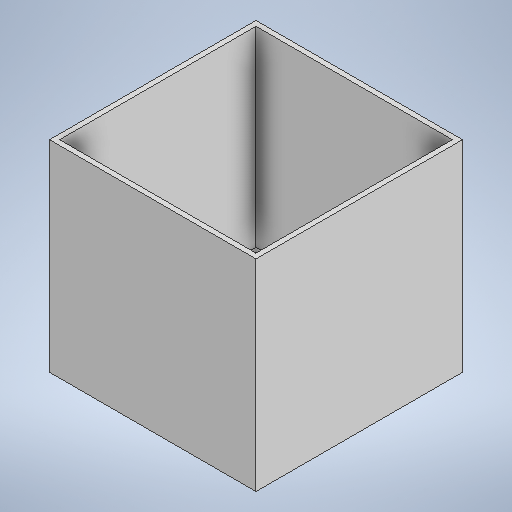
# Autodesk Inventor part: vaso
Saved by Autodesk Inventor 2025.1 (Build 291241000, 241)
## iProperties
Created: 2024-11-12
Part Number: vaso
Material: Genérico
Document SubType Name: Modeling
Designer: pedro
Density: 1 g/cm^3
Appearance: Padrão
Author: pedro
Autodesk Inventor part; units mm, degrees
ref_plane "YZ Plane" through (0, 0, 0) normal (1, 0, 0) x (0, 1, 0)
ref_plane "XZ Plane" through (0, 0, 0) normal (0, 1, 0) x (-1, 0, 0)
ref_plane "XY Plane" through (0, 0, 0) normal (0, 0, 1) x (1, 0, 0)
sketch "Esboço1" plane through (0, 0, 0) normal (0, 1, 0) x (-1, 0, 0)
  line L0 (102.5, 102.5) -> (-102.5, 102.5)
  line L1 (-102.5, 102.5) -> (-102.5, -102.5)
  line L2 (-102.5, -102.5) -> (102.5, -102.5)
  line L3 (102.5, -102.5) -> (102.5, 102.5)
  point P0 (0, 0)
  dimension "d0" = 205
  dimension "d1" = 205
  dimension "d2" = 102.5
  dimension "d3" = 102.5
  constraints: 8 end point, 2 parallel, 1 horizontal, 1 perpendicular
  measures "d0" distance of L2.end L1.end
  measures "d1" distance of L1.end L0.end
  measures "d2" distance from line of point (0, 0) L0
  measures "d3" distance from line of L3 point (0, 0)
extrude "Extrusão1" add sketch "Esboço1" along normal blind 200
sketch "Esboço2" plane through (0, 200, 0) normal (0, 1, 0) x (1, 0, 0)
  line L0 (-97.5, 97.5) -> (-97.5, -97.5)
  line L1 (-97.5, -97.5) -> (97.5, -97.5)
  line L2 (-97.5, 97.5) -> (97.5, 97.5)
  line L3 (97.5, 97.5) -> (97.5, -97.5)
  line L4 (-102.5, 102.5) -> (-102.5, -102.5) projected
  line L5 (102.5, 102.5) -> (-102.5, 102.5) projected
  line L6 (-102.5, -102.5) -> (102.5, -102.5) projected
  line L7 (102.5, -102.5) -> (102.5, 102.5) projected
  point P0 (0, 0)
  dimension "d6" = 5
  dimension "d7" = 5
  dimension "d8" = 5
  dimension "d9" = 5
  constraints: 8 end point, 2 perpendicular, 1 horizontal, 1 vertical
  measures "d6" distance between parallel lines of L4 L0
  measures "d7" distance between parallel lines of L5 L2
  measures "d8" distance between parallel lines of L6 L1
  measures "d9" distance between parallel lines of L7 L3
extrude "Extrusão2" cut sketch "Esboço2" against normal blind 190 contours L2 L3 L1 L0
